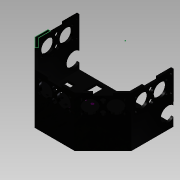
# Autodesk Inventor part: Kepala
Saved by Autodesk Inventor 2015 SP1 (Build 190203100, 203)
## iProperties
Created: 2015-02-01
Part Number: Kepala
Material: Generic
Document SubType Name: Modeling
Designer: Rafi Kurnia Putra
Density: 1 g/cm^3
Appearance: Smooth - Purple
Mass: 71.957 g
Surface Area: 473.113 cm^2
Volume: 71.957 cm^3
Author: Rafi Kurnia Putra
Autodesk Inventor part; units mm, degrees
ref_plane "YZ Plane" through (0, 0, 0) normal (1, 0, 0) x (0, 1, 0)
ref_plane "XZ Plane" through (0, 0, 0) normal (0, 1, 0) x (-1, 0, 0)
ref_plane "XY Plane" through (0, 0, 0) normal (0, 0, 1) x (1, 0, 0)
sketch "Sketch1" plane through (0, 0, 0) normal (0, 1, 0) x (-1, 0, 0)
  line L0 (60.406, -52.6639) -> (25.0211, -88.0488)
  line L1 (60.406, -52.6639) -> (60.406, 0)
  line L2 (-60.4057, -52.6639) -> (-60.4057, 0)
  line L3 (25.0211, -88.0488) -> (-25.0207, -88.0488)
  line L4 (-60.4057, 0) -> (60.406, 0)
  line L5 (-25.0207, -88.0488) -> (-60.4057, -52.6639)
  line L6 (57.406, 0) -> (57.406, -51.4212)
  line L7 (57.406, -51.4212) -> (23.7784, -85.0488)
  line L8 (23.7784, -85.0488) -> (-23.7781, -85.0488)
  line L9 (-23.7781, -85.0488) -> (-57.4057, -51.4212)
  line L10 (-57.4057, -51.4212) -> (-57.4057, 0)
  point P0 (0, -6165561.8884)
  point P1 (0, 0)
  point P2 (0.0002, 0)
  dimension "d195" = 120.8117
  dimension "d198" = 50.0418
  dimension "d199" = 50.0418
  dimension "d200" = 50.0418
  dimension "d201" = 52.6639
  dimension "d202" = 52.6639
  dimension "d204" = 3
  dimension "d205" = 51.4212
  dimension "d206" = 47.5566
  dimension "d207" = 47.5566
  dimension "d208" = 47.5566
  dimension "d209" = 51.4212
  dimension "d210" = 135
  dimension "d211" = 135
  dimension "d212" = 135
  dimension "d213" = 135
  dimension "d214" = 135
  dimension "d215" = 135
  dimension "d216" = 135
  dimension "d217" = 135
  dimension "d218" = 3
  dimension "d219" = 3
  dimension "d220" = 3
  constraints: 22 end point, 2 point on line, 1 horizontal, 1 horizontal alignment, 1 midpoint, 1 vertical, 3 other
  measures "d195" distance between parallel lines of L2 L1
  measures "d198" distance of L0.end L3.end
  measures "d199" distance of L0.start L0.end
  measures "d200" distance of L3.end L2.start
  measures "d201" distance of L0.start L1.end
  measures "d202" distance of L2.start L2.end
  measures "d204" distance between parallel lines of L6 L1
  measures "d205" distance of L6.start L6.end
  measures "d206" distance of L6.end L7.end
  measures "d207" distance of L7.end L8.end
  measures "d208" distance of L8.end L9.end
  measures "d209" distance of L9.end L10.end
  measures "d210" angle of L7 L6
  measures "d211" angle of L8 L7
  measures "d212" angle of L9 L8
  measures "d213" angle of L10 L9
  measures "d214" angle of L0 L1
  measures "d215" angle of L3 L0
  measures "d216" angle of L5 L3
  measures "d217" angle of L2 L5
  measures "d218" distance between parallel lines of L7 L0
  measures "d219" distance between parallel lines of L8 L3
  measures "d220" distance between parallel lines of L5 L9
extrude "Extrusion8" add sketch "Sketch1" along normal blind 3
extrude "Extrusion9" add sketch "Sketch1" against normal blind 60 contours L0 L3 L5 L2 L4 L10 L9 L8 L7 L6 L1
sketch "Sketch10" plane through (0, 3, 0) normal (0, 1, 0) x (1, 0, 0)
  circle A0 centre (13.2193, 36.61) radius 1.75
  circle A1 centre (39.7053, 36.61) radius 1.75
  circle A2 centre (39.7053, 12.2) radius 1.75
  circle A3 centre (13.2193, 12.2) radius 1.75
  circle A4 centre (20, 57.8773) radius 1.75
  circle A5 centre (-20, 57.8773) radius 1.75
  point P0 (0, 0)
  dimension "d115" = 3.5
  dimension "d116" = 3.5
  dimension "d117" = 3.5
  dimension "d118" = 3.5
  dimension "d119" = 3.5
  dimension "d120" = 3.5
  constraints: 6 centre point, 1 coincident
  measures "d115" diameter of A0
  measures "d116" diameter of A1
  measures "d117" diameter of A2
  measures "d118" diameter of A3
  measures "d119" diameter of A4
  measures "d120" diameter of A5
extrude "Extrusion10" cut sketch "Sketch10" against normal up to next
sketch "Sketch11" plane through (0, 3, 0) normal (0, 1, 0) x (1, 0, 0)
  line L0 (53.5557, 36.3929) -> (43.5557, 36.3929)
  line L1 (43.5557, 36.3929) -> (43.5557, 18.8929)
  line L2 (43.5557, 18.8929) -> (53.5557, 18.8929)
  line L3 (53.5557, 18.8929) -> (53.5557, 36.3929)
  line L4 (53.5557, 36.3929) -> (43.5557, 18.8929) construction
  line L5 (43.5557, 36.3929) -> (53.5557, 18.8929) construction
  line L6 (-53.5557, 36.3929) -> (-43.5557, 36.3929)
  line L7 (-43.5557, 36.3929) -> (-43.5557, 18.8929)
  line L8 (-43.5557, 18.8929) -> (-53.5557, 18.8929)
  line L9 (-53.5557, 18.8929) -> (-53.5557, 36.3929)
  line L10 (-53.5557, 36.3929) -> (-43.5557, 18.8929) construction
  line L11 (-43.5557, 36.3929) -> (-53.5557, 18.8929) construction
  line L12 (-8.75, 82.4488) -> (8.75, 82.4488)
  line L13 (8.75, 82.4488) -> (8.75, 67.4488)
  line L14 (8.75, 67.4488) -> (-8.75, 67.4488)
  line L15 (-8.75, 67.4488) -> (-8.75, 82.4488)
  line L16 (-8.75, 82.4488) -> (8.75, 67.4488) construction
  line L17 (8.75, 82.4488) -> (-8.75, 67.4488) construction
  line L18 (36.9856, 52.2544) -> (24.6113, 64.6288)
  line L19 (24.6113, 64.6288) -> (31.6823, 71.6998)
  line L20 (31.6823, 71.6998) -> (44.0567, 59.3254)
  line L21 (44.0567, 59.3254) -> (36.9856, 52.2544)
  line L22 (36.9856, 52.2544) -> (31.6823, 71.6998) construction
  line L23 (24.6113, 64.6288) -> (44.0567, 59.3254) construction
  line L24 (-44.057, 59.3254) -> (-31.6827, 71.6998)
  line L25 (-31.6827, 71.6998) -> (-24.6116, 64.6288)
  line L26 (-24.6116, 64.6288) -> (-36.986, 52.2544)
  line L27 (-36.986, 52.2544) -> (-44.057, 59.3254)
  line L28 (-44.057, 59.3254) -> (-24.6116, 64.6288) construction
  line L29 (-31.6827, 71.6998) -> (-36.986, 52.2544) construction
  line L30 (-23.7595, 81.9564) -> (-54.3136, 51.4023)
  line L31 (-23.7595, 81.9564) -> (-24.9616, 83.1585)
  line L32 (-54.3136, 51.4023) -> (-55.5157, 52.6044)
  line L33 (-24.9616, 83.1585) -> (-54.3136, 51.4023)
  line L34 (-55.5157, 52.6044) -> (-23.7595, 81.9564)
  line L35 (-39.6376, 67.2804) -> (60.3624, 67.2804) construction
  line L36 (-55.206, 49.2479) -> (-55.206, 6.0379)
  line L37 (21.6048, 82.8488) -> (-21.6052, 82.8488)
  line L38 (54.3133, 51.4023) -> (23.7592, 81.9564)
  line L39 (55.2057, 6.0379) -> (55.2057, 49.2479)
  point P0 (0, 0)
  point P1 (48.5557, 27.6429)
  point P2 (-48.5557, 27.6429)
  point P3 (0, 74.9488)
  point P4 (-2.6515, 135.1442)
  point P5 (34.334, 61.9771)
  point P6 (-34.3343, 61.9771)
  point P7 (-34.3343, 61.9771)
extrude "Extrusion11" cut sketch "Sketch11" against normal up to next contours L3 L2 L1 L0 | L6 L7 L8 L9 | L12 L13 L14 L15 | L18 L19 L20 L21 | L24 L25 L26 L27
sketch "Sketch12" plane through (0, 3, 0) normal (0, 1, 0) x (1, 0, 0)
  circle A0 centre (-37.593, 41.7496) radius 1.75 projected
  circle A1 centre (37.593, 41.7496) radius 1.75 projected
  point P0 (0, 0)
extrude "Extrusion12" cut sketch "Sketch12" against normal up to next
sketch "Sketch18" plane through (0, 0, 0) normal (0, -1, 0) x (1, 0, 0)
  circle A0 centre (49.9057, -48.3146) radius 1.75
  circle A1 centre (-49.906, -48.3146) radius 1.75
  line L0 (-56.906, -51.2141) -> (-56.906, 0) projected
  line L1 (-23.5713, -84.5488) -> (-56.906, -51.2141) projected
  line L2 (56.9057, 0) -> (56.9057, -51.2141) projected
  line L3 (56.9057, -51.2141) -> (23.571, -84.5488) projected
  point P0 (0, 0)
  dimension "d161" = 3.5
  dimension "d162" = 3.5
  dimension "d163" = 7
  dimension "d164" = 7
  dimension "d165" = 7
  dimension "d166" = 7
  constraints: 2 centre point
  measures "d161" diameter of A0
  measures "d162" diameter of A1
  measures "d163" distance from line of L1 A1.centre
  measures "d164" distance from line of A1.centre L0
  measures "d165" distance from line of A0.centre L2
  measures "d166" distance from line of L3 A0.centre
extrude "Extrusion19" cut sketch "Sketch18" against normal up to next
sketch "Sketch20" plane through (60.4057, 3, 0) normal (1, 0, 0) x (0, 0, -1)
  circle A0 centre (3, -59.0338) radius 1 projected
  circle A1 centre (3, -38.0338) radius 1 projected
  point P0 (0, -3)
extrude "Extrusion22" cut sketch "Sketch20" against normal through all
sketch "Sketch21" plane through (0, 3, 0) normal (0, 1, 0) x (1, 0, 0)
  line L0 (-24.65, 5.9273) -> (-24.65, 25.8273)
  line L1 (-29.55, 7.4273) -> (-29.55, 25.8273)
  line L2 (-24.65, 25.8273) -> (-29.55, 25.8273)
  line L3 (-24.65, 5.9273) -> (-29.55, 5.9273)
  line L4 (-29.55, 5.9273) -> (-29.55, 7.4273)
  line L5 (-22.2, 3.7546) -> (-32, 3.7546)
  line L6 (-32, 3.7546) -> (-32, 28)
  line L7 (-32, 28) -> (-22.2, 28)
  line L8 (-22.2, 28) -> (-22.2, 3.7546)
  line L9 (-22.2, 3.7546) -> (-32, 28) construction
  line L10 (-32, 3.7546) -> (-22.2, 28) construction
  point P0 (0, 0)
  point P1 (-27.1, 15.8773)
  constraints: 22 end point, 3 horizontal, 2 midpoint, 2 parallel, 2 perpendicular
extrude "Extrusion23" cut sketch "Sketch21" against normal up to next contours L3 L4 L1 L2 L0 | L5 L6 L7 L8
sketch "Sketch22" plane through (0, -60, 0) normal (0, -1, 0) x (1, 0, 0)
  line L0 (57.406, -36.3929) -> (60.406, -36.3929)
  line L1 (57.406, -18.8928) -> (60.406, -18.8929)
  line L2 (57.406, -18.8928) -> (60.406, -18.8928) construction
  line L3 (60.406, -18.8929) -> (60.406, -36.3929)
  line L4 (57.406, -36.3929) -> (57.406, -18.8928)
  line L5 (34.4047, -74.4222) -> (36.526, -76.5435)
  line L6 (46.7791, -62.0478) -> (48.9004, -64.1691)
  line L7 (36.526, -76.5435) -> (48.9004, -64.1691)
  line L8 (46.7791, -62.0478) -> (34.4047, -74.4222)
  line L9 (-8.7498, -88.0488) -> (-8.7498, -85.0488)
  line L10 (0, 0) -> (0, -8)
  line L11 (-57.406, -36.3929) -> (-60.406, -36.3929)
  line L12 (-57.406, -18.8928) -> (-60.406, -18.8929)
  line L13 (-57.406, -18.8928) -> (-60.406, -18.8928) construction
  line L14 (-60.406, -18.8929) -> (-60.406, -36.3929)
  line L15 (-57.406, -36.3929) -> (-57.406, -18.8928)
  line L16 (-34.4047, -74.4222) -> (-36.526, -76.5435)
  line L17 (-46.7791, -62.0478) -> (-48.9004, -64.1691)
  line L18 (-36.526, -76.5435) -> (-48.9004, -64.1691)
  line L19 (-46.7791, -62.0478) -> (-34.4047, -74.4222)
  line L20 (8.7498, -88.0488) -> (8.7498, -85.0488)
  line L21 (-57.406, 0) -> (-60.406, 0) projected
  line L22 (-60.406, 0) -> (-60.406, -52.6639) projected
  line L23 (-60.406, -52.6639) -> (-25.0211, -88.0488) projected
  line L24 (-25.0211, -88.0488) -> (25.0207, -88.0488) projected
  line L25 (25.0207, -88.0488) -> (60.4057, -52.6639) projected
  line L26 (60.4057, -52.6639) -> (60.4057, 0) projected
  line L27 (60.4057, 0) -> (57.4057, 0) projected
  line L28 (57.4057, 0) -> (57.4057, -51.4212) projected
  line L29 (57.4057, -51.4212) -> (23.7781, -85.0488) projected
  line L30 (23.7781, -85.0488) -> (-23.7784, -85.0488) projected
  line L31 (-23.7784, -85.0488) -> (-57.406, -51.4212) projected
  line L32 (-57.406, -51.4212) -> (-57.406, 0) projected
  line L33 (-60.406, 0) -> (-60.406, -52.6639) projected
  line L34 (60.4057, -52.6639) -> (60.4057, 0) projected
  line L35 (23.7781, -85.0488) -> (-23.7784, -85.0488) projected
  line L36 (8.7498, -88.0488) -> (-8.7498, -88.0488)
  line L37 (8.7498, -85.0488) -> (-8.7498, -85.0488)
  line L38 (36.9856, -52.2544) -> (44.0567, -59.3254) projected
  line L39 (31.6823, -71.6998) -> (24.6113, -64.6288) projected
  line L40 (53.5557, -36.3929) -> (43.5557, -36.3929) projected
  line L41 (-43.5557, -36.3929) -> (-53.5557, -36.3929) projected
  point P0 (-0.0002, -87)
  dimension "d181" = 17.5
  dimension "d221" = 3
  dimension "d222" = 0
  dimension "d223" = 17.5001
  dimension "d225" = 3
  dimension "d231" = 0
  constraints: 46 end point, 11 symmetric about line, 5 collinear, 3 horizontal, 2 parallel, 1 equal length, 1 horizontal alignment, 1 perpendicular, 1 other
  measures "d181" distance of L12.end L11.end
  measures "d221" distance between parallel lines of L14 L15
  measures "d222" distance from line of L22 L11.end
  measures "d223" distance of L1.start L0.start
  measures "d225" distance of L16.start L16.end
  measures "d231" distance between parallel lines of L36 L24
sketch "Sketch23" plane through (0, 3, 0) normal (0, 1, 0) x (1, 0, 0)
  circle A0 centre (-27.94, 46.62) radius 1.75 projected
  circle A1 centre (43, 59.9982) radius 1.75 projected
  circle A2 centre (-27.94, 46.62) radius 1.5875 projected
  circle A3 centre (20.32, 40.27) radius 1.5875 projected
  point P0 (0, 0)
extrude "Extrusion27" cut sketch "Sketch23" against normal up to next contours A2 | A3
sketch "Sketch26" plane through (25.0207, 3, -88.0488) normal (0, 0, -1) x (-1, 0, 0)
  line L0 (14.0407, -9.138) -> (36.0007, -9.138) projected
  line L1 (36.0007, -4.158) -> (14.0407, -4.158) projected
  line L2 (36.5007, -8.638) -> (36.5007, -4.658) projected
  line L3 (13.5407, -4.658) -> (13.5407, -8.638) projected
  arc A0 (13.5407, -8.638) -> (14.0407, -9.138) centre (14.0407, -8.638) ccw projected
  arc A1 (36.0007, -9.138) -> (36.5007, -8.638) centre (36.0007, -8.638) ccw projected
  arc A2 (36.5007, -4.658) -> (36.0007, -4.158) centre (36.0007, -4.658) ccw projected
  arc A3 (14.0407, -4.158) -> (13.5407, -4.658) centre (14.0407, -4.658) ccw projected
  line L4 (14.0407, -2) -> (36.0007, -2)
  arc A4 (38.6587, -4.658) -> (36.0007, -2) centre (36.0007, -4.658) ccw
  line L5 (38.6587, -4.658) -> (38.6587, -8.638)
  arc A5 (36.0007, -11.296) -> (38.6587, -8.638) centre (36.0007, -8.638) ccw
  line L6 (36.0007, -11.296) -> (14.0407, -11.296)
  arc A6 (11.3827, -8.638) -> (14.0407, -11.296) centre (14.0407, -8.638) ccw
  line L7 (11.3827, -8.638) -> (11.3827, -4.658)
  arc A7 (14.0407, -2) -> (11.3827, -4.658) centre (14.0407, -4.658) ccw
  point P0 (25.0207, -3)
  constraints: 8 end point, 8 point on circle, 4 centre point, 7 other
extrude "Extrusion30" [suppressed]
extrude "Extrusion31" cut sketch "Sketch22" against normal blind 3 contours L4 L1 L3 L0 | L6 L7 L5 L8 | L20 L24 L9 L30 | L16 L18 L17 L19 | L11 L14 L12 L15
sketch "Sketch27" plane through (-60.406, -60, -52.6639) normal (-0.7071068, 0, -0.7071068) x (-0.7071068, 0, 0.7071068)
  line L0 (-33.7712, 3) -> (-16.2712, 3) projected
  line L1 (-16.2712, 0) -> (-16.2712, 3) projected
  line L2 (-33.7712, 0) -> (-33.7712, 3) projected
  line L3 (0, 0) -> (-50.0418, 0) projected
  point P0 (-5.4745, 60)
extrude "Extrusion32" cut sketch "Sketch27" against normal blind 3
sketch "Sketch28" plane through (57.406, -60, -18.8928) normal (1, 0, 0) x (0, 0, -1)
  line L0 (17.5001, 0) -> (0, 0) projected
  line L1 (17.5001, 0) -> (17.5001, 3) projected
  line L2 (17.5001, 3) -> (0, 3) projected
  line L3 (0, 0) -> (0, 3) projected
  point P0 (-18.8928, 60)
extrude "Extrusion33" cut sketch "Sketch28" along normal mid plane 3
sketch "Sketch31" plane through (0, 3, 0) normal (0, 1, 0) x (1, 0, 0)
  circle A0 centre (20.32, 40.27) radius 1.5875 projected
  circle A1 centre (20.32, 40.27) radius 1.75
  circle A2 centre (37.593, 41.7496) radius 1.75 projected
  circle A3 centre (-27.94, 46.62) radius 1.5875 projected
  circle A4 centre (-27.94, 46.62) radius 1.5875 projected
  circle A5 centre (-27.94, 46.62) radius 1.75
  point P0 (0, 0)
  dimension "d242" = 3.5
  dimension "d243" = 3.5
  constraints: 2 centre point, 2 coincident
  measures "d242" diameter of A1
  measures "d243" diameter of A5
extrude "Extrusion36" cut sketch "Sketch31" against normal up to next contours A1 | A5
sketch "Sketch34" plane through (25.0207, 3, -88.0488) normal (0, 0, -1) x (-1, 0, 0)
  circle A0 centre (36.4509, -47.6838) radius 8.5 projected
  circle A1 centre (13.5909, -47.6838) radius 8.5 projected
  circle A2 centre (25.0209, -41.1438) radius 3 projected
  circle A3 centre (5.9369, -40.0298) radius 1.6 projected
  circle A4 centre (5.9369, -55.3378) radius 1.6 projected
  circle A5 centre (25.0209, -54.2238) radius 3 projected
  circle A6 centre (44.1049, -55.3378) radius 1.6 projected
  circle A7 centre (44.1049, -40.0298) radius 1.6 projected
  point P0 (25.0207, -3)
extrude "Extrusion40" cut sketch "Sketch34" against normal up to next
sketch "Sketch35" plane through (25.0207, -60, -88.0488) normal (0.7071068, 0, -0.7071068) x (-0.7071068, 0, -0.7071068)
  circle A0 centre (-36.4509, 15.3162) radius 8.5 projected
  circle A1 centre (-13.5909, 15.3162) radius 8.5 projected
  circle A2 centre (-25.0209, 21.8562) radius 3 projected
  circle A3 centre (-25.0209, 8.7762) radius 3 projected
  circle A4 centre (-44.1049, 22.9702) radius 1.6 projected
  circle A5 centre (-44.1049, 7.6622) radius 1.6 projected
  circle A6 centre (-5.9369, 7.6622) radius 1.6 projected
  circle A7 centre (-5.9369, 22.9702) radius 1.6 projected
  point P0 (-44.5675, 60)
extrude "Extrusion41" cut sketch "Sketch35" against normal up to next
sketch "Sketch36" plane through (60.4057, 3, 0) normal (1, 0, 0) x (0, 0, -1)
  circle A0 centre (39.0729, -47.6838) radius 8.5 projected
  circle A1 centre (16.2129, -47.6838) radius 8.5 projected
  circle A2 centre (27.6429, -41.1438) radius 3 projected
  circle A3 centre (27.6429, -54.2238) radius 3 projected
  circle A4 centre (8.5589, -55.3378) radius 1.6 projected
  circle A5 centre (8.5589, -40.0298) radius 1.6 projected
  circle A6 centre (46.7269, -40.0298) radius 1.6 projected
  circle A7 centre (46.7269, -55.3378) radius 1.6 projected
  point P0 (0, -3)
extrude "Extrusion42" cut sketch "Sketch36" against normal blind 180
sketch "Sketch37" plane through (-60.406, -60, -52.6639) normal (-0.7071068, 0, -0.7071068) x (-0.7071068, 0, 0.7071068)
  circle A0 centre (-13.5909, 15.3162) radius 8.5 projected
  circle A1 centre (-36.4509, 15.3162) radius 8.5 projected
  circle A2 centre (-25.0209, 21.8562) radius 3 projected
  circle A3 centre (-25.0209, 8.7762) radius 3 projected
  circle A4 centre (-44.1049, 7.6622) radius 1.6 projected
  circle A5 centre (-44.1049, 22.9702) radius 1.6 projected
  circle A6 centre (-5.9369, 22.9702) radius 1.6 projected
  circle A7 centre (-5.9369, 7.6622) radius 1.6 projected
  point P0 (-5.4745, 60)
extrude "Extrusion43" cut sketch "Sketch37" against normal up to next
sketch "Sketch38" plane through (60.4057, 3, 0) normal (1, 0, 0) x (0, 0, -1)
  circle A0 centre (6.7939, -16.9) radius 9.2 projected
  point P0 (0, -3)
extrude "Extrusion44" cut sketch "Sketch38" against normal through all
sketch "Sketch40" plane through (0, 0, 0) normal (0, -1, 0) x (1, 0, 0)
  circle A0 centre (12, -46) radius 1.75
  circle A1 centre (12, -29) radius 1.75
  circle A2 centre (21, -46) radius 1.75
  circle A3 centre (21, -29) radius 1.75
  line L0 (0, -56) -> (0, -18) construction
  circle A4 centre (-12, -46) radius 1.75
  circle A5 centre (-12, -29) radius 1.75
  circle A6 centre (-21, -46) radius 1.75
  circle A7 centre (-21, -29) radius 1.75
  point P0 (0, 0)
  dimension "d262" = 3.5
  dimension "d263" = 3.5
  dimension "d264" = 3.5
  dimension "d265" = 3.5
  constraints: 8 centre point, 4 symmetric about line, 2 end point, 1 vertical, 4 other
  measures "d262" diameter of A0
  measures "d263" diameter of A1
  measures "d264" diameter of A2
  measures "d265" diameter of A3
extrude "Extrusion45" cut sketch "Sketch40" against normal through all
sketch "Sketch41" plane through (0, -60, 0) normal (0, -1, 0) x (1, 0, 0)
  line L0 (-48.9006, -64.1693) -> (-46.7792, -62.048) projected
  line L1 (-46.7792, -62.048) -> (-57.406, -51.4212) projected
  line L2 (-57.406, -51.4212) -> (-57.406, -36.3929) projected
  line L3 (-57.406, -36.3929) -> (-60.406, -36.3929) projected
  line L4 (-60.406, -36.3929) -> (-60.406, -52.6639) projected
  line L5 (-60.406, -52.6639) -> (-48.9006, -64.1693) projected
  point P0 (0, 0)
body "Solid2"
